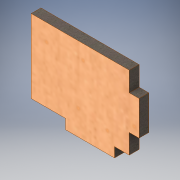
# Autodesk Inventor part: Limiter3
Saved by Autodesk Inventor 2019 (Build 230136000, 136)
## iProperties
Created: 2021-01-03
Part Number: Limiter3
Material: Дерево (вишня)
Document SubType Name: Modeling
Designer: Professional
Density: 0.63 g/cm^3
Appearance: Вишневое дерево — натуральный — со слабым глянцем
Author: Professional
Autodesk Inventor part; units mm, degrees
ref_plane "YZ Plane" through (0, 0, 0) normal (1, 0, 0) x (0, 1, 0)
ref_plane "XZ Plane" through (0, 0, 0) normal (0, 1, 0) x (-1, 0, 0)
ref_plane "XY Plane" through (0, 0, 0) normal (0, 0, 1) x (1, 0, 0)
sketch "Эскиз1" plane through (0, 0, 0) normal (0, 0, 1) x (1, 0, 0)
  line L0 (0, 0) -> (-20, 0)
  line L1 (-20, 0) -> (-20, 4)
  line L2 (-20, 4) -> (-34, 4)
  line L3 (-34, 4) -> (-34, 34)
  line L4 (-34, 34) -> (6, 34)
  line L5 (6, 34) -> (6, 26)
  line L6 (6, 26) -> (10, 26)
  line L7 (10, 26) -> (10, 12)
  line L8 (10, 12) -> (6, 12)
  line L9 (6, 12) -> (6, 4)
  line L10 (0, 4) -> (0, 0)
  line L11 (0, 4) -> (6, 4)
  dimension "d0" = 4
  dimension "d1" = 30
  dimension "d2" = 14
  dimension "d4" = 20
  dimension "d5" = 14
  dimension "d6" = 6
  constraints: 24 end point, 8 perpendicular, 4 point on line, 2 equal length, 1 horizontal, 1 parallel
  measures "d0" distance of L0.end L1.end
  measures "d1" distance between parallel lines of L2 L4
  measures "d2" distance between parallel lines of L8 L6
  measures "d4" distance of L0.start L0.end
  measures "d5" distance between parallel lines of L1 L3
  measures "d6" distance between parallel lines of L9 L10
extrude "Выдавливание1" add sketch "Эскиз1" along normal blind 4
